Autodesk Inventor part; units mm, degrees
(part 2 of 3)
sketch "Sketch4" plane through (0, 0, -2.75) normal (0, 0, -1) x (-1, 0, 0)
  arc A0 (0.3991, 3.7387) -> (0.581, 3.8546) centre (0.3991, 3.9394) ccw
  line L0 (0.581, 3.8546) -> (0.7391, 4.1936)
  arc A1 (1.0847, 4.3585) -> (0.7391, 4.1936) centre (1.012, 4.0663) ccw
  arc A2 (1.2398, 4.317) -> (1.0847, 4.3585) centre (0, 0) ccw
  arc A3 (1.4567, 4.0013) -> (1.2398, 4.317) centre (1.1567, 4.0275) ccw
  line L1 (1.4567, 4.0013) -> (1.4241, 3.6287)
  arc A4 (1.4241, 3.6287) -> (1.5237, 3.4373) centre (1.6241, 3.6112) ccw
  line L2 (1.5237, 3.4373) -> (2.2149, 3.0382)
  arc A5 (2.2149, 3.0382) -> (2.4305, 3.0476) centre (2.3153, 3.2121) ccw
  line L3 (2.4305, 3.0476) -> (2.7369, 3.2622)
  arc A6 (3.1187, 3.2322) -> (2.7369, 3.2622) centre (2.9096, 3.0155) ccw
  arc A7 (3.2322, 3.1187) -> (3.1187, 3.2322) centre (0, 0) ccw
  arc A8 (3.2622, 2.7369) -> (3.2322, 3.1187) centre (3.0155, 2.9096) ccw
  line L4 (3.2622, 2.7369) -> (3.0476, 2.4305)
  arc A9 (3.0476, 2.4305) -> (3.0382, 2.2149) centre (3.2121, 2.3153) ccw
  line L5 (3.0382, 2.2149) -> (3.4373, 1.5237)
  arc A10 (3.4373, 1.5237) -> (3.6287, 1.4241) centre (3.6112, 1.6241) ccw
  line L6 (3.6287, 1.4241) -> (4.0013, 1.4567)
  arc A11 (4.317, 1.2398) -> (4.0013, 1.4567) centre (4.0275, 1.1567) ccw
  arc A12 (4.3585, 1.0847) -> (4.317, 1.2398) centre (0, 0) ccw
  arc A13 (4.1936, 0.7391) -> (4.3585, 1.0847) centre (4.0663, 1.012) ccw
  line L7 (4.1936, 0.7391) -> (3.8546, 0.581)
  arc A14 (3.8546, 0.581) -> (3.7387, 0.3991) centre (3.9394, 0.3991) ccw
  line L8 (3.7387, 0.3991) -> (3.7387, -0.3991)
  arc A15 (3.7387, -0.3991) -> (3.8546, -0.581) centre (3.9394, -0.3991) ccw
  line L9 (3.8546, -0.581) -> (4.1936, -0.7391)
  arc A16 (4.3585, -1.0847) -> (4.1936, -0.7391) centre (4.0663, -1.012) ccw
  arc A17 (4.317, -1.2398) -> (4.3585, -1.0847) centre (0, 0) ccw
  arc A18 (4.0013, -1.4567) -> (4.317, -1.2398) centre (4.0275, -1.1567) ccw
  line L10 (4.0013, -1.4567) -> (3.6287, -1.4241)
  arc A19 (3.6287, -1.4241) -> (3.4373, -1.5237) centre (3.6112, -1.6241) ccw
  line L11 (3.4373, -1.5237) -> (3.0382, -2.2149)
  arc A20 (3.0382, -2.2149) -> (3.0476, -2.4305) centre (3.2121, -2.3153) ccw
  line L12 (3.0476, -2.4305) -> (3.2622, -2.7369)
  arc A21 (3.2322, -3.1187) -> (3.2622, -2.7369) centre (3.0155, -2.9096) ccw
  arc A22 (3.1187, -3.2322) -> (3.2322, -3.1187) centre (0, 0) ccw
  arc A23 (2.7369, -3.2622) -> (3.1187, -3.2322) centre (2.9096, -3.0155) ccw
  line L13 (2.7369, -3.2622) -> (2.4305, -3.0476)
  arc A24 (2.4305, -3.0476) -> (2.2149, -3.0382) centre (2.3153, -3.2121) ccw
  line L14 (2.2149, -3.0382) -> (1.5237, -3.4373)
  arc A25 (1.5237, -3.4373) -> (1.4241, -3.6287) centre (1.6241, -3.6112) ccw
  line L15 (1.4241, -3.6287) -> (1.4567, -4.0013)
  arc A26 (1.2398, -4.317) -> (1.4567, -4.0013) centre (1.1567, -4.0275) ccw
  arc A27 (1.0847, -4.3585) -> (1.2398, -4.317) centre (0, 0) ccw
  arc A28 (0.7391, -4.1936) -> (1.0847, -4.3585) centre (1.012, -4.0663) ccw
  line L16 (0.7391, -4.1936) -> (0.581, -3.8546)
  arc A29 (0.581, -3.8546) -> (0.3991, -3.7387) centre (0.3991, -3.9394) ccw
  line L17 (0.3991, -3.7387) -> (-0.3991, -3.7387)
  arc A30 (-0.3991, -3.7387) -> (-0.581, -3.8546) centre (-0.3991, -3.9394) ccw
  line L18 (-0.581, -3.8546) -> (-0.7391, -4.1936)
  arc A31 (-1.0847, -4.3585) -> (-0.7391, -4.1936) centre (-1.012, -4.0663) ccw
  arc A32 (-1.2398, -4.317) -> (-1.0847, -4.3585) centre (0, 0) ccw
  arc A33 (-1.4567, -4.0013) -> (-1.2398, -4.317) centre (-1.1567, -4.0275) ccw
  line L19 (-1.4567, -4.0013) -> (-1.4241, -3.6287)
  arc A34 (-1.4241, -3.6287) -> (-1.5237, -3.4373) centre (-1.6241, -3.6112) ccw
  line L20 (-1.5237, -3.4373) -> (-2.2149, -3.0382)
  arc A35 (-2.2149, -3.0382) -> (-2.4305, -3.0476) centre (-2.3153, -3.2121) ccw
  line L21 (-2.4305, -3.0476) -> (-2.7369, -3.2622)
  arc A36 (-3.1187, -3.2322) -> (-2.7369, -3.2622) centre (-2.9096, -3.0155) ccw
  arc A37 (-3.2322, -3.1187) -> (-3.1187, -3.2322) centre (0, 0) ccw
  arc A38 (-3.2622, -2.7369) -> (-3.2322, -3.1187) centre (-3.0155, -2.9096) ccw
  line L22 (-3.2622, -2.7369) -> (-3.0476, -2.4305)
  arc A39 (-3.0476, -2.4305) -> (-3.0382, -2.2149) centre (-3.2121, -2.3153) ccw
  line L23 (-3.0382, -2.2149) -> (-3.4373, -1.5237)
  arc A40 (-3.4373, -1.5237) -> (-3.6287, -1.4241) centre (-3.6112, -1.6241) ccw
  line L24 (-3.6287, -1.4241) -> (-4.0013, -1.4567)
  arc A41 (-4.317, -1.2398) -> (-4.0013, -1.4567) centre (-4.0275, -1.1567) ccw
  arc A42 (-4.3585, -1.0847) -> (-4.317, -1.2398) centre (0, 0) ccw
  arc A43 (-4.1936, -0.7391) -> (-4.3585, -1.0847) centre (-4.0663, -1.012) ccw
  line L25 (-4.1936, -0.7391) -> (-3.8546, -0.581)
  arc A44 (-3.8546, -0.581) -> (-3.7387, -0.3991) centre (-3.9394, -0.3991) ccw
  line L26 (-3.7387, -0.3991) -> (-3.7387, 0.3991)
  arc A45 (-3.7387, 0.3991) -> (-3.8546, 0.581) centre (-3.9394, 0.3991) ccw
  line L27 (-3.8546, 0.581) -> (-4.1936, 0.7391)
  arc A46 (-4.3585, 1.0847) -> (-4.1936, 0.7391) centre (-4.0663, 1.012) ccw
  arc A47 (-4.317, 1.2398) -> (-4.3585, 1.0847) centre (0, 0) ccw
  arc A48 (-4.0013, 1.4567) -> (-4.317, 1.2398) centre (-4.0275, 1.1567) ccw
  line L28 (-4.0013, 1.4567) -> (-3.6287, 1.4241)
  arc A49 (-3.6287, 1.4241) -> (-3.4373, 1.5237) centre (-3.6112, 1.6241) ccw
  line L29 (-3.4373, 1.5237) -> (-3.0382, 2.2149)
  arc A50 (-3.0382, 2.2149) -> (-3.0476, 2.4305) centre (-3.2121, 2.3153) ccw
  line L30 (-3.0476, 2.4305) -> (-3.2622, 2.7369)
  arc A51 (-3.2322, 3.1187) -> (-3.2622, 2.7369) centre (-3.0155, 2.9096) ccw
  arc A52 (-3.1187, 3.2322) -> (-3.2322, 3.1187) centre (0, 0) ccw
  arc A53 (-2.7369, 3.2622) -> (-3.1187, 3.2322) centre (-2.9096, 3.0155) ccw
  line L31 (-2.7369, 3.2622) -> (-2.4305, 3.0476)
  arc A54 (-2.4305, 3.0476) -> (-2.2149, 3.0382) centre (-2.3153, 3.2121) ccw
  line L32 (-2.2149, 3.0382) -> (-1.5237, 3.4373)
  arc A55 (-1.5237, 3.4373) -> (-1.4241, 3.6287) centre (-1.6241, 3.6112) ccw
  line L33 (-1.4241, 3.6287) -> (-1.4567, 4.0013)
  arc A56 (-1.2398, 4.317) -> (-1.4567, 4.0013) centre (-1.1567, 4.0275) ccw
  arc A57 (-1.0847, 4.3585) -> (-1.2398, 4.317) centre (0, 0) ccw
  arc A58 (-0.7391, 4.1936) -> (-1.0847, 4.3585) centre (-1.012, 4.0663) ccw
  line L34 (-0.7391, 4.1936) -> (-0.581, 3.8546)
  arc A59 (-0.581, 3.8546) -> (-0.3991, 3.7387) centre (-0.3991, 3.9394) ccw
  line L35 (-0.3991, 3.7387) -> (0.3991, 3.7387)
  circle A60 centre (0, 0) radius 6.84
  arc A61 (3.6199, -1.5237) -> (3.5239, -1.5737) centre (3.6112, -1.6241) ccw
  circle A62 centre (0, 0) radius 4.4915 construction
  line L36 (-2.3024, -3.1898) -> (-1.6112, -3.5889)
  arc A63 (-1.5984, -3.6134) -> (-1.6112, -3.5889) centre (-1.6241, -3.6112) ccw
  line L37 (-1.5984, -3.6134) -> (-1.631, -3.986)
  arc A64 (-1.631, -3.986) -> (-1.2882, -4.4852) centre (-1.1567, -4.0275) ccw
  arc A65 (-1.2882, -4.4852) -> (-1.127, -4.5283) centre (0, 0) ccw
  arc A66 (-1.127, -4.5283) -> (-0.5805, -4.2675) centre (-1.012, -4.0663) ccw
  line L38 (-0.5805, -4.2675) -> (-0.4224, -3.9285)
  arc A67 (-0.3991, -3.9137) -> (-0.4224, -3.9285) centre (-0.3991, -3.9394) ccw
  line L39 (-0.3991, -3.9137) -> (0.3991, -3.9137)
  arc A68 (0.4224, -3.9285) -> (0.3991, -3.9137) centre (0.3991, -3.9394) ccw
  line L40 (0.4224, -3.9285) -> (0.5805, -4.2675)
  arc A69 (0.5805, -4.2675) -> (1.127, -4.5283) centre (1.012, -4.0663) ccw
  arc A70 (1.127, -4.5283) -> (1.2882, -4.4852) centre (0, 0) ccw
  arc A71 (1.2882, -4.4852) -> (1.631, -3.986) centre (1.1567, -4.0275) ccw
  line L41 (1.631, -3.986) -> (1.5984, -3.6134)
  arc A72 (1.6112, -3.5889) -> (1.5984, -3.6134) centre (1.6241, -3.6112) ccw
  line L42 (1.6112, -3.5889) -> (2.3024, -3.1898)
  arc A73 (2.3301, -3.191) -> (2.3024, -3.1898) centre (2.3153, -3.2121) ccw
  line L43 (2.3301, -3.191) -> (2.6365, -3.4055)
  arc A74 (2.6365, -3.4055) -> (3.2402, -3.3582) centre (2.9096, -3.0155) ccw
  arc A75 (3.2402, -3.3582) -> (3.3582, -3.2402) centre (0, 0) ccw
  arc A76 (3.3582, -3.2402) -> (3.4055, -2.6365) centre (3.0155, -2.9096) ccw
  line L44 (3.4055, -2.6365) -> (3.191, -2.3301)
  arc A77 (3.1898, -2.3024) -> (3.191, -2.3301) centre (3.2121, -2.3153) ccw
  line L45 (3.1898, -2.3024) -> (3.5889, -1.6112)
  arc A78 (3.6134, -1.5984) -> (3.5889, -1.6112) centre (3.6112, -1.6241) ccw
  line L46 (3.6134, -1.5984) -> (3.986, -1.631)
  arc A79 (3.986, -1.631) -> (4.4852, -1.2882) centre (4.0275, -1.1567) ccw
  arc A80 (4.4852, -1.2882) -> (4.5283, -1.127) centre (0, 0) ccw
  arc A81 (4.5283, -1.127) -> (4.2675, -0.5805) centre (4.0663, -1.012) ccw
  line L47 (4.2675, -0.5805) -> (3.9285, -0.4224)
  arc A82 (3.9137, -0.3991) -> (3.9285, -0.4224) centre (3.9394, -0.3991) ccw
  line L48 (3.9137, -0.3991) -> (3.9137, 0.3991)
  arc A83 (3.9285, 0.4224) -> (3.9137, 0.3991) centre (3.9394, 0.3991) ccw
  line L49 (3.9285, 0.4224) -> (4.2675, 0.5805)
  arc A84 (4.2675, 0.5805) -> (4.5283, 1.127) centre (4.0663, 1.012) ccw
  arc A85 (4.5283, 1.127) -> (4.4852, 1.2882) centre (0, 0) ccw
  arc A86 (4.4852, 1.2882) -> (3.986, 1.631) centre (4.0275, 1.1567) ccw
  line L50 (3.986, 1.631) -> (3.6134, 1.5984)
  arc A87 (3.5889, 1.6112) -> (3.6134, 1.5984) centre (3.6112, 1.6241) ccw
  line L51 (3.5889, 1.6112) -> (3.1898, 2.3024)
  arc A88 (3.191, 2.3301) -> (3.1898, 2.3024) centre (3.2121, 2.3153) ccw
  line L52 (3.191, 2.3301) -> (3.4055, 2.6365)
  arc A89 (3.4055, 2.6365) -> (3.3582, 3.2402) centre (3.0155, 2.9096) ccw
  arc A90 (3.3582, 3.2402) -> (3.2402, 3.3582) centre (0, 0) ccw
  arc A91 (3.2402, 3.3582) -> (2.6365, 3.4055) centre (2.9096, 3.0155) ccw
  line L53 (2.6365, 3.4055) -> (2.3301, 3.191)
  arc A92 (2.3024, 3.1898) -> (2.3301, 3.191) centre (2.3153, 3.2121) ccw
  line L54 (2.3024, 3.1898) -> (1.6112, 3.5889)
  arc A93 (1.5984, 3.6134) -> (1.6112, 3.5889) centre (1.6241, 3.6112) ccw
  line L55 (1.5984, 3.6134) -> (1.631, 3.986)
  arc A94 (1.631, 3.986) -> (1.2882, 4.4852) centre (1.1567, 4.0275) ccw
  arc A95 (1.2882, 4.4852) -> (1.127, 4.5283) centre (0, 0) ccw
  arc A96 (1.127, 4.5283) -> (0.5805, 4.2675) centre (1.012, 4.0663) ccw
  line L56 (0.5805, 4.2675) -> (0.4224, 3.9285)
  arc A97 (0.3991, 3.9137) -> (0.4224, 3.9285) centre (0.3991, 3.9394) ccw
  line L57 (0.3991, 3.9137) -> (-0.3991, 3.9137)
  arc A98 (-0.4224, 3.9285) -> (-0.3991, 3.9137) centre (-0.3991, 3.9394) ccw
  line L58 (-0.4224, 3.9285) -> (-0.5805, 4.2675)
  arc A99 (-0.5805, 4.2675) -> (-1.127, 4.5283) centre (-1.012, 4.0663) ccw
  arc A100 (-1.127, 4.5283) -> (-1.2882, 4.4852) centre (0, 0) ccw
  arc A101 (-1.2882, 4.4852) -> (-1.631, 3.986) centre (-1.1567, 4.0275) ccw
  line L59 (-1.631, 3.986) -> (-1.5984, 3.6134)
  arc A102 (-1.6112, 3.5889) -> (-1.5984, 3.6134) centre (-1.6241, 3.6112) ccw
  line L60 (-1.6112, 3.5889) -> (-2.3024, 3.1898)
  arc A103 (-2.3301, 3.191) -> (-2.3024, 3.1898) centre (-2.3153, 3.2121) ccw
  line L61 (-2.3301, 3.191) -> (-2.6365, 3.4055)
  arc A104 (-2.6365, 3.4055) -> (-3.2402, 3.3582) centre (-2.9096, 3.0155) ccw
  arc A105 (-3.2402, 3.3582) -> (-3.3582, 3.2402) centre (0, 0) ccw
  arc A106 (-3.3582, 3.2402) -> (-3.4055, 2.6365) centre (-3.0155, 2.9096) ccw
  line L62 (-3.4055, 2.6365) -> (-3.191, 2.3301)
  arc A107 (-3.1898, 2.3024) -> (-3.191, 2.3301) centre (-3.2121, 2.3153) ccw
  line L63 (-3.1898, 2.3024) -> (-3.5889, 1.6112)
  arc A108 (-3.6134, 1.5984) -> (-3.5889, 1.6112) centre (-3.6112, 1.6241) ccw
  line L64 (-3.6134, 1.5984) -> (-3.986, 1.631)
  arc A109 (-3.986, 1.631) -> (-4.4852, 1.2882) centre (-4.0275, 1.1567) ccw
  arc A110 (-4.4852, 1.2882) -> (-4.5283, 1.127) centre (0, 0) ccw
  arc A111 (-4.5283, 1.127) -> (-4.2675, 0.5805) centre (-4.0663, 1.012) ccw
  line L65 (-4.2675, 0.5805) -> (-3.9285, 0.4224)
  arc A112 (-3.9137, 0.3991) -> (-3.9285, 0.4224) centre (-3.9394, 0.3991) ccw
  line L66 (-3.9137, 0.3991) -> (-3.9137, -0.3991)
  arc A113 (-3.9285, -0.4224) -> (-3.9137, -0.3991) centre (-3.9394, -0.3991) ccw
  line L67 (-3.9285, -0.4224) -> (-4.2675, -0.5805)
  arc A114 (-4.2675, -0.5805) -> (-4.5283, -1.127) centre (-4.0663, -1.012) ccw
  arc A115 (-4.5283, -1.127) -> (-4.4852, -1.2882) centre (0, 0) ccw
  arc A116 (-4.4852, -1.2882) -> (-3.986, -1.631) centre (-4.0275, -1.1567) ccw
  line L68 (-3.986, -1.631) -> (-3.6134, -1.5984)
  arc A117 (-3.5889, -1.6112) -> (-3.6134, -1.5984) centre (-3.6112, -1.6241) ccw
  line L69 (-3.5889, -1.6112) -> (-3.1898, -2.3024)
  arc A118 (-3.191, -2.3301) -> (-3.1898, -2.3024) centre (-3.2121, -2.3153) ccw
  line L70 (-3.191, -2.3301) -> (-3.4055, -2.6365)
  arc A119 (-3.4055, -2.6365) -> (-3.3582, -3.2402) centre (-3.0155, -2.9096) ccw
  arc A120 (-3.3582, -3.2402) -> (-3.2402, -3.3582) centre (0, 0) ccw
  arc A121 (-3.2402, -3.3582) -> (-2.6365, -3.4055) centre (-2.9096, -3.0155) ccw
  line L71 (-2.6365, -3.4055) -> (-2.3301, -3.191)
  arc A122 (-2.3024, -3.1898) -> (-2.3301, -3.191) centre (-2.3153, -3.2121) ccw
  dimension "d0" = 28.6479
  dimension "d1" = 0.3
  dimension "d2" = 0.75
  dimension "d3" = 50
  dimension "d4" = 1.05
  dimension "d74" = 8.983
  dimension "d34" = 13.68
  dimension "d75" = 0.175
  constraints: 242 point on circle, 144 end point, 122 centre point, 3 coincident, 98 other
  measures "d34" diameter of A60
  measures "d75" distance between parallel lines of L20 L36
sketch "HTD3M 33Teeth" plane through (0, 0, 0) normal (0, 0, 1) x (1, 0, 0)
  arc A0 (15.2288, 2.1154) -> (15.2079, 2.2607) centre (0, 0) ccw
  arc A1 (15.1485, 1.9322) -> (15.2288, 2.1154) centre (15.0396, 2.0891) ccw
  line L0 (15.1485, 1.9322) -> (14.5361, 1.5072)
  arc A2 (14.5361, 1.5072) -> (14.1386, 0.7015) centre (15.0646, 0.7456) ccw
  line L1 (14.1386, 0.7015) -> (14.1413, 0.6456)
  arc A3 (14.1413, 0.6456) -> (14.6135, -0.1187) centre (15.0672, 0.6897) ccw
  line L2 (14.6135, -0.1187) -> (15.2636, -0.4835)
  arc A4 (15.3609, -0.6583) -> (15.2636, -0.4835) centre (15.1701, -0.6501) ccw
  arc A5 (15.3539, -0.8049) -> (15.3609, -0.6583) centre (0, 0) ccw
  arc A6 (15.2404, -0.9696) -> (15.3539, -0.8049) centre (15.1632, -0.7949) ccw
  line L3 (15.2404, -0.9696) -> (14.5586, -1.271)
  arc A7 (14.5586, -1.271) -> (14.0159, -1.9869) centre (14.9335, -2.1188) ccw
  line L4 (14.0159, -1.9869) -> (14.0079, -2.0423)
  arc A8 (14.0079, -2.0423) -> (14.327, -2.8821) centre (14.9255, -2.1742) ccw
  line L5 (14.327, -2.8821) -> (14.8962, -3.3634)
  arc A9 (14.9587, -3.5534) -> (14.8962, -3.3634) centre (14.7729, -3.5093) ccw
  arc A10 (14.9241, -3.6961) -> (14.9587, -3.5534) centre (0, 0) ccw
  arc A11 (14.7815, -3.8363) -> (14.9241, -3.6961) centre (14.7387, -3.6502) ccw
  line L6 (14.7815, -3.8363) -> (14.055, -4.0033)
  arc A12 (14.055, -4.0033) -> (13.3866, -4.6035) centre (14.2626, -4.9067) ccw
  line L7 (13.3866, -4.6035) -> (13.3683, -4.6564)
  arc A13 (13.3683, -4.6564) -> (13.5226, -5.5415) centre (14.2443, -4.9596) ccw
  line L8 (13.5226, -5.5415) -> (13.9905, -6.1218)
  arc A14 (14.0159, -6.3202) -> (13.9905, -6.1218) centre (13.8418, -6.2417) ccw
  arc A15 (13.9549, -6.4537) -> (14.0159, -6.3202) centre (0, 0) ccw
  arc A16 (13.7884, -6.5644) -> (13.9549, -6.4537) centre (13.7816, -6.3735) ccw
  line L9 (13.7884, -6.5644) -> (13.0434, -6.5908)
  arc A17 (13.0434, -6.5908) -> (12.2735, -7.0538) centre (13.0763, -7.5173) ccw
  line L10 (12.2735, -7.0538) -> (12.2455, -7.1022)
  arc A18 (12.2455, -7.1022) -> (12.2295, -8.0005) centre (13.0483, -7.5657) ccw
  line L11 (12.2295, -8.0005) -> (12.5791, -8.6589)
  arc A19 (12.5665, -8.8585) -> (12.5791, -8.6589) centre (12.4104, -8.7484) ccw
  arc A20 (12.4814, -8.9781) -> (12.5665, -8.8585) centre (0, 0) ccw
  arc A21 (12.2969, -9.0552) -> (12.4814, -8.9781) centre (12.3263, -8.8665) ccw
  line L12 (12.2969, -9.0552) -> (11.5604, -8.9402)
  arc A22 (11.5604, -8.9402) -> (10.7167, -9.249) centre (11.4173, -9.8561) ccw
  line L13 (10.7167, -9.249) -> (10.6801, -9.2914)
  arc A23 (10.6801, -9.2914) -> (10.4944, -10.1704) centre (11.3806, -9.8984) ccw
  line L14 (10.4944, -10.1704) -> (10.7131, -10.883)
  arc A24 (10.663, -11.0766) -> (10.7131, -10.883) centre (10.5305, -10.939) ccw
  arc A25 (10.5567, -11.1779) -> (10.663, -11.0766) centre (0, 0) ccw
  arc A26 (10.3609, -11.2188) -> (10.5567, -11.1779) centre (10.4256, -11.0391) ccw
  line L15 (10.3609, -11.2188) -> (9.6595, -10.9665)
  arc A27 (9.6595, -10.9665) -> (8.7727, -11.1101) centre (9.3457, -11.8387) ccw
  line L16 (8.7727, -11.1101) -> (8.7286, -11.1447)
  arc A28 (8.7286, -11.1447) -> (8.38, -11.9726) centre (9.3017, -11.8733) ccw
  line L17 (8.38, -11.9726) -> (8.4599, -12.7138)
  arc A29 (8.374, -12.8944) -> (8.4599, -12.7138) centre (8.27, -12.7343) ccw
  arc A30 (8.2505, -12.9738) -> (8.374, -12.8944) centre (0, 0) ccw
  arc A31 (8.0505, -12.9769) -> (8.2505, -12.9738) centre (8.148, -12.8126) ccw
  line L18 (8.0505, -12.9769) -> (7.4095, -12.5963)
  arc A32 (7.4095, -12.5963) -> (6.5115, -12.5695) centre (6.9363, -13.3935) ccw
  line L19 (6.5115, -12.5695) -> (6.4618, -12.5952)
  arc A33 (6.4618, -12.5952) -> (5.9627, -13.3422) centre (6.8865, -13.4191) ccw
  line L20 (5.9627, -13.3422) -> (5.9009, -14.0851)
  arc A34 (5.7824, -14.2462) -> (5.9009, -14.0851) centre (5.7105, -14.0692) ccw
  arc A35 (5.6461, -14.3008) -> (5.7824, -14.2462) centre (0, 0) ccw
  arc A36 (5.4492, -14.2659) -> (5.6461, -14.3008) centre (5.576, -14.1231) ccw
  line L21 (5.4492, -14.2659) -> (4.8917, -13.771)
  arc A37 (4.8917, -13.771) -> (4.0151, -13.5747) centre (4.2762, -14.4641) ccw
  line L22 (4.0151, -13.5747) -> (3.9613, -13.5905)
  arc A38 (3.9613, -13.5905) -> (3.33, -14.2296) centre (4.2225, -14.4799) ccw
  line L23 (3.33, -14.2296) -> (3.1286, -14.9473)
  arc A39 (2.9818, -15.0831) -> (3.1286, -14.9473) centre (2.9447, -14.8957) ccw
  arc A40 (2.8376, -15.1109) -> (2.9818, -15.0831) centre (0, 0) ccw
  arc A41 (2.6508, -15.0394) -> (2.8376, -15.1109) centre (2.8024, -14.9232) ccw
  line L24 (2.6508, -15.0394) -> (2.1972, -14.4479)
  arc A42 (2.1972, -14.4479) -> (1.3735, -14.0892) centre (1.4616, -15.012) ccw
  line L25 (1.3735, -14.0892) -> (1.3177, -14.0946)
  arc A43 (1.3177, -14.0946) -> (0.5768, -14.6026) centre (1.4059, -15.0174) ccw
  line L26 (0.5768, -14.6026) -> (0.2433, -15.2693)
  arc A44 (0.0734, -15.3748) -> (0.2433, -15.2693) centre (0.0725, -15.1838) ccw
  arc A45 (-0.0734, -15.3748) -> (0.0734, -15.3748) centre (0, 0) ccw
  arc A46 (-0.2433, -15.2693) -> (-0.0734, -15.3748) centre (-0.0725, -15.1838) ccw
  line L27 (-0.2433, -15.2693) -> (-0.5768, -14.6026)
  arc A47 (-0.5768, -14.6026) -> (-1.3177, -14.0946) centre (-1.4059, -15.0174) ccw
  line L28 (-1.3177, -14.0946) -> (-1.3735, -14.0892)
  arc A48 (-1.3735, -14.0892) -> (-2.1972, -14.4479) centre (-1.4616, -15.012) ccw
  line L29 (-2.1972, -14.4479) -> (-2.6508, -15.0394)
  arc A49 (-2.8376, -15.1109) -> (-2.6508, -15.0394) centre (-2.8024, -14.9232) ccw
  arc A50 (-2.9818, -15.0831) -> (-2.8376, -15.1109) centre (0, 0) ccw
  arc A51 (-3.1286, -14.9473) -> (-2.9818, -15.0831) centre (-2.9447, -14.8957) ccw
  line L30 (-3.1286, -14.9473) -> (-3.33, -14.2296)
  arc A52 (-3.33, -14.2296) -> (-3.9613, -13.5905) centre (-4.2225, -14.4799) ccw
  line L31 (-3.9613, -13.5905) -> (-4.0151, -13.5747)
  arc A53 (-4.0151, -13.5747) -> (-4.8917, -13.771) centre (-4.2762, -14.4641) ccw
  line L32 (-4.8917, -13.771) -> (-5.4492, -14.2659)
  arc A54 (-5.6461, -14.3008) -> (-5.4492, -14.2659) centre (-5.576, -14.1231) ccw
  arc A55 (-5.7824, -14.2462) -> (-5.6461, -14.3008) centre (0, 0) ccw
  arc A56 (-5.9009, -14.0851) -> (-5.7824, -14.2462) centre (-5.7105, -14.0692) ccw
  line L33 (-5.9009, -14.0851) -> (-5.9627, -13.3422)
  arc A57 (-5.9627, -13.3422) -> (-6.4618, -12.5952) centre (-6.8865, -13.4191) ccw
  line L34 (-6.4618, -12.5952) -> (-6.5115, -12.5695)
  arc A58 (-6.5115, -12.5695) -> (-7.4095, -12.5963) centre (-6.9363, -13.3935) ccw
  line L35 (-7.4095, -12.5963) -> (-8.0505, -12.9769)
  arc A59 (-8.2505, -12.9738) -> (-8.0505, -12.9769) centre (-8.148, -12.8126) ccw
  arc A60 (-8.374, -12.8944) -> (-8.2505, -12.9738) centre (0, 0) ccw
  arc A61 (-8.4599, -12.7138) -> (-8.374, -12.8944) centre (-8.27, -12.7343) ccw
  line L36 (-8.4599, -12.7138) -> (-8.38, -11.9726)
  arc A62 (-8.38, -11.9726) -> (-8.7286, -11.1447) centre (-9.3017, -11.8733) ccw
  line L37 (-8.7286, -11.1447) -> (-8.7727, -11.1101)
  arc A63 (-8.7727, -11.1101) -> (-9.6595, -10.9665) centre (-9.3457, -11.8387) ccw
  line L38 (-9.6595, -10.9665) -> (-10.3609, -11.2188)
  arc A64 (-10.5567, -11.1779) -> (-10.3609, -11.2188) centre (-10.4256, -11.0391) ccw
  arc A65 (-10.663, -11.0766) -> (-10.5567, -11.1779) centre (0, 0) ccw
  arc A66 (-10.7131, -10.883) -> (-10.663, -11.0766) centre (-10.5305, -10.939) ccw
  line L39 (-10.7131, -10.883) -> (-10.4944, -10.1704)
  arc A67 (-10.4944, -10.1704) -> (-10.6801, -9.2914) centre (-11.3806, -9.8984) ccw
  line L40 (-10.6801, -9.2914) -> (-10.7167, -9.249)
  arc A68 (-10.7167, -9.249) -> (-11.5604, -8.9402) centre (-11.4173, -9.8561) ccw
  line L41 (-11.5604, -8.9402) -> (-12.2969, -9.0552)
  arc A69 (-12.4814, -8.9781) -> (-12.2969, -9.0552) centre (-12.3263, -8.8665) ccw
  arc A70 (-12.5665, -8.8585) -> (-12.4814, -8.9781) centre (0, 0) ccw
  arc A71 (-12.5791, -8.6589) -> (-12.5665, -8.8585) centre (-12.4104, -8.7484) ccw
  line L42 (-12.5791, -8.6589) -> (-12.2295, -8.0005)
  arc A72 (-12.2295, -8.0005) -> (-12.2455, -7.1022) centre (-13.0483, -7.5657) ccw
  line L43 (-12.2455, -7.1022) -> (-12.2735, -7.0538)
  arc A73 (-12.2735, -7.0538) -> (-13.0434, -6.5908) centre (-13.0763, -7.5173) ccw
  line L44 (-13.0434, -6.5908) -> (-13.7884, -6.5644)
  arc A74 (-13.9549, -6.4537) -> (-13.7884, -6.5644) centre (-13.7816, -6.3735) ccw
  arc A75 (-14.0159, -6.3202) -> (-13.9549, -6.4537) centre (0, 0) ccw
  arc A76 (-13.9905, -6.1218) -> (-14.0159, -6.3202) centre (-13.8418, -6.2417) ccw
  line L45 (-13.9905, -6.1218) -> (-13.5226, -5.5415)
  arc A77 (-13.5226, -5.5415) -> (-13.3683, -4.6564) centre (-14.2443, -4.9596) ccw
  line L46 (-13.3683, -4.6564) -> (-13.3866, -4.6035)
  arc A78 (-13.3866, -4.6035) -> (-14.055, -4.0033) centre (-14.2626, -4.9067) ccw
  line L47 (-14.055, -4.0033) -> (-14.7815, -3.8363)
  arc A79 (-14.9241, -3.6961) -> (-14.7815, -3.8363) centre (-14.7387, -3.6502) ccw
  arc A80 (-14.9587, -3.5534) -> (-14.9241, -3.6961) centre (0, 0) ccw
  arc A81 (-14.8962, -3.3634) -> (-14.9587, -3.5534) centre (-14.7729, -3.5093) ccw
  line L48 (-14.8962, -3.3634) -> (-14.327, -2.8821)
  arc A82 (-14.327, -2.8821) -> (-14.0079, -2.0423) centre (-14.9255, -2.1742) ccw
  line L49 (-14.0079, -2.0423) -> (-14.0159, -1.9869)
  arc A83 (-14.0159, -1.9869) -> (-14.5586, -1.271) centre (-14.9335, -2.1188) ccw
  line L50 (-14.5586, -1.271) -> (-15.2404, -0.9696)
  arc A84 (-15.3539, -0.8049) -> (-15.2404, -0.9696) centre (-15.1632, -0.7949) ccw
  arc A85 (-15.3609, -0.6583) -> (-15.3539, -0.8049) centre (0, 0) ccw
  arc A86 (-15.2636, -0.4835) -> (-15.3609, -0.6583) centre (-15.1701, -0.6501) ccw
  line L51 (-15.2636, -0.4835) -> (-14.6135, -0.1187)
  arc A87 (-14.6135, -0.1187) -> (-14.1413, 0.6456) centre (-15.0672, 0.6897) ccw
  line L52 (-14.1413, 0.6456) -> (-14.1386, 0.7015)
  arc A88 (-14.1386, 0.7015) -> (-14.5361, 1.5072) centre (-15.0646, 0.7456) ccw
  line L53 (-14.5361, 1.5072) -> (-15.1485, 1.9322)
  arc A89 (-15.2288, 2.1154) -> (-15.1485, 1.9322) centre (-15.0396, 2.0891) ccw
  arc A90 (-15.2079, 2.2607) -> (-15.2288, 2.1154) centre (0, 0) ccw
  arc A91 (-15.0792, 2.4139) -> (-15.2079, 2.2607) centre (-15.019, 2.2326) ccw
  line L54 (-15.0792, 2.4139) -> (-14.3719, 2.6491)
  arc A92 (-14.3719, 2.6491) -> (-13.7636, 3.3102) centre (-14.6644, 3.5287) ccw
  line L55 (-13.7636, 3.3102) -> (-13.7504, 3.3646)
  arc A93 (-13.7504, 3.3646) -> (-13.9881, 4.231) centre (-14.6512, 3.5832) ccw
  line L56 (-13.9881, 4.231) -> (-14.5091, 4.7642)
  arc A94 (-14.5532, 4.9593) -> (-14.5091, 4.7642) centre (-14.3724, 4.8977) ccw
  arc A95 (-14.5052, 5.098) -> (-14.5532, 4.9593) centre (0, 0) ccw
  arc A96 (-14.3499, 5.224) -> (-14.5052, 5.098) centre (-14.325, 5.0346) ccw
  line L57 (-14.3499, 5.224) -> (-13.6108, 5.3211)
  arc A97 (-13.6108, 5.3211) -> (-12.8884, 5.8551) centre (-13.7316, 6.2402) ccw
  line L58 (-12.8884, 5.8551) -> (-12.8651, 5.9061)
  arc A98 (-12.8651, 5.9061) -> (-12.9346, 6.8018) centre (-13.7083, 6.2912) ccw
  line L59 (-12.9346, 6.8018) -> (-13.3452, 7.4239)
  arc A99 (-13.3517, 7.6239) -> (-13.3452, 7.4239) centre (-13.1858, 7.5291) ccw
  arc A100 (-13.2783, 7.751) -> (-13.3517, 7.6239) centre (0, 0) ccw
  arc A101 (-13.1019, 7.8453) -> (-13.2783, 7.751) centre (-13.1133, 7.6547) ccw
  line L60 (-13.1019, 7.8453) -> (-12.3578, 7.8008)
  arc A102 (-12.3578, 7.8008) -> (-11.5474, 8.1885) centre (-12.3025, 8.7262) ccw
  line L61 (-11.5474, 8.1885) -> (-11.5149, 8.2341)
  arc A103 (-11.5149, 8.2341) -> (-11.4137, 9.1267) centre (-12.27, 8.7718) ccw
  line L62 (-11.4137, 9.1267) -> (-11.6991, 9.8154)
  arc A104 (-11.6676, 10.0129) -> (-11.6991, 9.8154) centre (-11.5226, 9.8885) ccw
  arc A105 (-11.5715, 10.1238) -> (-11.6676, 10.0129) centre (0, 0) ccw
  arc A106 (-11.3804, 10.1831) -> (-11.5715, 10.1238) centre (-11.4277, 9.9981) ccw
  line L63 (-11.3804, 10.1831) -> (-10.6582, 9.9986)
  arc A107 (-10.6582, 9.9986) -> (-9.789, 10.2259) centre (-10.4287, 10.8968) ccw
  line L64 (-9.789, 10.2259) -> (-9.7485, 10.2645)
  arc A108 (-9.7485, 10.2645) -> (-9.4801, 11.1219) centre (-10.3882, 10.9354) ccw
  line L65 (-9.4801, 11.1219) -> (-9.6301, 11.8521)
  arc A109 (-9.5618, 12.0401) -> (-9.6301, 11.8521) centre (-9.443, 11.8905) ccw
  arc A110 (-9.4464, 12.1308) -> (-9.5618, 12.0401) centre (0, 0) ccw
  arc A111 (-9.2476, 12.1529) -> (-9.4464, 12.1308) centre (-9.329, 11.9801) ccw
  line L66 (-9.2476, 12.1529) -> (-8.5733, 11.835)
  arc A112 (-8.5733, 11.835) -> (-7.6769, 11.8936) centre (-8.178, 12.6735) ccw
  line L67 (-7.6769, 11.8936) -> (-7.6298, 11.9239)
  arc A113 (-7.6298, 11.9239) -> (-7.204, 12.715) centre (-8.1309, 12.7038) ccw
  line L68 (-7.204, 12.715) -> (-7.213, 13.4604)
  arc A114 (-7.1104, 13.6321) -> (-7.213, 13.4604) centre (-7.0221, 13.4627) ccw
  arc A115 (-6.9799, 13.6993) -> (-7.1104, 13.6321) centre (0, 0) ccw
  arc A116 (-6.7805, 13.6834) -> (-6.9799, 13.6993) centre (-6.8932, 13.5291) ccw
  line L69 (-6.7805, 13.6834) -> (-6.1786, 13.2436)
  arc A117 (-6.1786, 13.2436) -> (-5.2872, 13.1316) centre (-5.6318, 13.9922) ccw
  line L70 (-5.2872, 13.1316) -> (-5.2353, 13.1524)
  arc A118 (-5.2353, 13.1524) -> (-4.6675, 13.8486) centre (-5.5798, 14.013) ccw
  line L71 (-4.6675, 13.8486) -> (-4.5353, 14.5822)
  arc A119 (-4.402, 14.7314) -> (-4.5353, 14.5822) centre (-4.3473, 14.5484) ccw
  arc A120 (-4.2612, 14.7727) -> (-4.402, 14.7314) centre (0, 0) ccw
  arc A121 (-4.0684, 14.7193) -> (-4.2612, 14.7727) centre (-4.2082, 14.5892) ccw
  line L72 (-4.0684, 14.7193) -> (-3.5606, 14.1736)
  arc A122 (-3.5606, 14.1736) -> (-2.7065, 13.8949) centre (-2.882, 14.8051) ccw
  line L73 (-2.7065, 13.8949) -> (-2.6515, 13.9055)
  arc A123 (-2.6515, 13.9055) -> (-1.9623, 14.4817) centre (-2.827, 14.8157) ccw
  line L74 (-1.9623, 14.4817) -> (-1.6936, 15.177)
  arc A124 (-1.5345, 15.2982) -> (-1.6936, 15.177) centre (-1.5155, 15.1082) ccw
  arc A125 (-1.3884, 15.3122) -> (-1.5345, 15.2982) centre (0, 0) ccw
  arc A126 (-1.2092, 15.2233) -> (-1.3884, 15.3122) centre (-1.3712, 15.122) ccw
  line L75 (-1.2092, 15.2233) -> (-0.8139, 14.5913)
  arc A127 (-0.8139, 14.5913) -> (-0.028, 14.156) centre (-0.028, 15.083) ccw
  line L76 (-0.028, 14.156) -> (0.028, 14.156)
  arc A128 (0.028, 14.156) -> (0.8139, 14.5913) centre (0.028, 15.083) ccw
  line L77 (0.8139, 14.5913) -> (1.2092, 15.2233)
  arc A129 (1.3884, 15.3122) -> (1.2092, 15.2233) centre (1.3712, 15.122) ccw
  arc A130 (1.5345, 15.2982) -> (1.3884, 15.3122) centre (0, 0) ccw
  arc A131 (1.6936, 15.177) -> (1.5345, 15.2982) centre (1.5155, 15.1082) ccw
  line L78 (1.6936, 15.177) -> (1.9623, 14.4817)
  arc A132 (1.9623, 14.4817) -> (2.6515, 13.9055) centre (2.827, 14.8157) ccw
  line L79 (2.6515, 13.9055) -> (2.7065, 13.8949)
  arc A133 (2.7065, 13.8949) -> (3.5606, 14.1736) centre (2.882, 14.8051) ccw
  line L80 (3.5606, 14.1736) -> (4.0684, 14.7193)
  arc A134 (4.2612, 14.7727) -> (4.0684, 14.7193) centre (4.2082, 14.5892) ccw
  arc A135 (4.402, 14.7314) -> (4.2612, 14.7727) centre (0, 0) ccw
  arc A136 (4.5353, 14.5822) -> (4.402, 14.7314) centre (4.3473, 14.5484) ccw
  line L81 (4.5353, 14.5822) -> (4.6675, 13.8486)
  arc A137 (4.6675, 13.8486) -> (5.2353, 13.1524) centre (5.5798, 14.013) ccw
  line L82 (5.2353, 13.1524) -> (5.2872, 13.1316)
  arc A138 (5.2872, 13.1316) -> (6.1786, 13.2436) centre (5.6318, 13.9922) ccw
  line L83 (6.1786, 13.2436) -> (6.7805, 13.6834)
  arc A139 (6.9799, 13.6993) -> (6.7805, 13.6834) centre (6.8932, 13.5291) ccw
  arc A140 (7.1104, 13.6321) -> (6.9799, 13.6993) centre (0, 0) ccw
  arc A141 (7.213, 13.4604) -> (7.1104, 13.6321) centre (7.0221, 13.4627) ccw
  line L84 (7.213, 13.4604) -> (7.204, 12.715)
  arc A142 (7.204, 12.715) -> (7.6298, 11.9239) centre (8.1309, 12.7038) ccw
  line L85 (7.6298, 11.9239) -> (7.6769, 11.8936)
  arc A143 (7.6769, 11.8936) -> (8.5733, 11.835) centre (8.178, 12.6735) ccw
  line L86 (8.5733, 11.835) -> (9.2476, 12.1529)
  arc A144 (9.4464, 12.1308) -> (9.2476, 12.1529) centre (9.329, 11.9801) ccw
  arc A145 (9.5618, 12.0401) -> (9.4464, 12.1308) centre (0, 0) ccw
  arc A146 (9.6301, 11.8521) -> (9.5618, 12.0401) centre (9.443, 11.8905) ccw
  line L87 (9.6301, 11.8521) -> (9.4801, 11.1219)
  arc A147 (9.4801, 11.1219) -> (9.7485, 10.2645) centre (10.3882, 10.9354) ccw
  line L88 (9.7485, 10.2645) -> (9.789, 10.2259)
  arc A148 (9.789, 10.2259) -> (10.6582, 9.9986) centre (10.4287, 10.8968) ccw
  line L89 (10.6582, 9.9986) -> (11.3804, 10.1831)
  arc A149 (11.5715, 10.1238) -> (11.3804, 10.1831) centre (11.4277, 9.9981) ccw
  arc A150 (11.6676, 10.0129) -> (11.5715, 10.1238) centre (0, 0) ccw
  arc A151 (11.6991, 9.8154) -> (11.6676, 10.0129) centre (11.5226, 9.8885) ccw
  line L90 (11.6991, 9.8154) -> (11.4137, 9.1267)
  arc A152 (11.4137, 9.1267) -> (11.5149, 8.2341) centre (12.27, 8.7718) ccw
  line L91 (11.5149, 8.2341) -> (11.5474, 8.1885)
  arc A153 (11.5474, 8.1885) -> (12.3578, 7.8008) centre (12.3025, 8.7262) ccw
  line L92 (12.3578, 7.8008) -> (13.1019, 7.8453)
  arc A154 (13.2783, 7.751) -> (13.1019, 7.8453) centre (13.1133, 7.6547) ccw
  arc A155 (13.3517, 7.6239) -> (13.2783, 7.751) centre (0, 0) ccw
  arc A156 (13.3452, 7.4239) -> (13.3517, 7.6239) centre (13.1858, 7.5291) ccw
  line L93 (13.3452, 7.4239) -> (12.9346, 6.8018)
  arc A157 (12.9346, 6.8018) -> (12.8651, 5.9061) centre (13.7083, 6.2912) ccw
  line L94 (12.8651, 5.9061) -> (12.8884, 5.8551)
  arc A158 (12.8884, 5.8551) -> (13.6108, 5.3211) centre (13.7316, 6.2402) ccw
  line L95 (13.6108, 5.3211) -> (14.3499, 5.224)
  arc A159 (14.5052, 5.098) -> (14.3499, 5.224) centre (14.325, 5.0346) ccw
  arc A160 (14.5532, 4.9593) -> (14.5052, 5.098) centre (0, 0) ccw
  arc A161 (14.5091, 4.7642) -> (14.5532, 4.9593) centre (14.3724, 4.8977) ccw
  line L96 (14.5091, 4.7642) -> (13.9881, 4.231)
  arc A162 (13.9881, 4.231) -> (13.7504, 3.3646) centre (14.6512, 3.5832) ccw
  line L97 (13.7504, 3.3646) -> (13.7636, 3.3102)
  arc A163 (13.7636, 3.3102) -> (14.3719, 2.6491) centre (14.6644, 3.5287) ccw
  line L98 (14.3719, 2.6491) -> (15.0792, 2.4139)
  arc A164 (15.2079, 2.2607) -> (15.0792, 2.4139) centre (15.019, 2.2326) ccw
  arc A165 (15.2288, 2.1154) -> (15.2079, 2.2607) centre (0, 0) ccw
  arc A166 (15.1485, 1.9322) -> (15.2288, 2.1154) centre (15.0396, 2.0891) ccw
  line L99 (15.1485, 1.9322) -> (14.5361, 1.5072)
  arc A167 (14.5361, 1.5072) -> (14.1386, 0.7015) centre (15.0646, 0.7456) ccw
  line L100 (14.1386, 0.7015) -> (14.1413, 0.6456)
  arc A168 (14.1413, 0.6456) -> (14.6135, -0.1187) centre (15.0672, 0.6897) ccw
  line L101 (14.6135, -0.1187) -> (15.2636, -0.4835)
  arc A169 (15.3609, -0.6583) -> (15.2636, -0.4835) centre (15.1701, -0.6501) ccw
  arc A170 (15.3539, -0.8049) -> (15.3609, -0.6583) centre (0, 0) ccw
  arc A171 (15.2404, -0.9696) -> (15.3539, -0.8049) centre (15.1632, -0.7949) ccw
  line L102 (15.2404, -0.9696) -> (14.5586, -1.271)
  arc A172 (14.5586, -1.271) -> (14.0159, -1.9869) centre (14.9335, -2.1188) ccw
  line L103 (14.0159, -1.9869) -> (14.0079, -2.0423)
  arc A173 (14.0079, -2.0423) -> (14.327, -2.8821) centre (14.9255, -2.1742) ccw
  line L104 (14.327, -2.8821) -> (14.8962, -3.3634)
  arc A174 (14.9587, -3.5534) -> (14.8962, -3.3634) centre (14.7729, -3.5093) ccw
  arc A175 (14.9241, -3.6961) -> (14.9587, -3.5534) centre (0, 0) ccw
  arc A176 (14.7815, -3.8363) -> (14.9241, -3.6961) centre (14.7387, -3.6502) ccw
  line L105 (14.7815, -3.8363) -> (14.055, -4.0033)
  arc A177 (14.055, -4.0033) -> (13.3866, -4.6035) centre (14.2626, -4.9067) ccw
  line L106 (13.3866, -4.6035) -> (13.3683, -4.6564)
  arc A178 (13.3683, -4.6564) -> (13.5226, -5.5415) centre (14.2443, -4.9596) ccw
  line L107 (13.5226, -5.5415) -> (13.9905, -6.1218)
  arc A179 (14.0159, -6.3202) -> (13.9905, -6.1218) centre (13.8418, -6.2417) ccw
  arc A180 (13.9549, -6.4537) -> (14.0159, -6.3202) centre (0, 0) ccw
  arc A181 (13.7884, -6.5644) -> (13.9549, -6.4537) centre (13.7816, -6.3735) ccw
  line L108 (13.7884, -6.5644) -> (13.0434, -6.5908)
  arc A182 (13.0434, -6.5908) -> (12.2735, -7.0538) centre (13.0763, -7.5173) ccw
  line L109 (12.2735, -7.0538) -> (12.2455, -7.1022)
  arc A183 (12.2455, -7.1022) -> (12.2295, -8.0005) centre (13.0483, -7.5657) ccw
  line L110 (12.2295, -8.0005) -> (12.5791, -8.6589)
  arc A184 (12.5665, -8.8585) -> (12.5791, -8.6589) centre (12.4104, -8.7484) ccw
  arc A185 (12.4814, -8.9781) -> (12.5665, -8.8585) centre (0, 0) ccw
  arc A186 (12.2969, -9.0552) -> (12.4814, -8.9781) centre (12.3263, -8.8665) ccw
  line L111 (12.2969, -9.0552) -> (11.5604, -8.9402)
  arc A187 (11.5604, -8.9402) -> (10.7167, -9.249) centre (11.4173, -9.8561) ccw
  line L112 (10.7167, -9.249) -> (10.6801, -9.2914)
  arc A188 (10.6801, -9.2914) -> (10.4944, -10.1704) centre (11.3806, -9.8984) ccw
  line L113 (10.4944, -10.1704) -> (10.7131, -10.883)
  arc A189 (10.663, -11.0766) -> (10.7131, -10.883) centre (10.5305, -10.939) ccw
  arc A190 (10.5567, -11.1779) -> (10.663, -11.0766) centre (0, 0) ccw
  arc A191 (10.3609, -11.2188) -> (10.5567, -11.1779) centre (10.4256, -11.0391) ccw
  line L114 (10.3609, -11.2188) -> (9.6595, -10.9665)
  arc A192 (9.6595, -10.9665) -> (8.7727, -11.1101) centre (9.3457, -11.8387) ccw
  line L115 (8.7727, -11.1101) -> (8.7286, -11.1447)
  arc A193 (8.7286, -11.1447) -> (8.38, -11.9726) centre (9.3017, -11.8733) ccw
  line L116 (8.38, -11.9726) -> (8.4599, -12.7138)
  arc A194 (8.374, -12.8944) -> (8.4599, -12.7138) centre (8.27, -12.7343) ccw
  arc A195 (8.2505, -12.9738) -> (8.374, -12.8944) centre (0, 0) ccw
  arc A196 (8.0505, -12.9769) -> (8.2505, -12.9738) centre (8.148, -12.8126) ccw
  line L117 (8.0505, -12.9769) -> (7.4095, -12.5963)
  arc A197 (7.4095, -12.5963) -> (6.5115, -12.5695) centre (6.9363, -13.3935) ccw
  line L118 (6.5115, -12.5695) -> (6.4618, -12.5952)
  arc A198 (6.4618, -12.5952) -> (5.9627, -13.3422) centre (6.8865, -13.4191) ccw
  line L119 (5.9627, -13.3422) -> (5.9009, -14.0851)
  arc A199 (5.7824, -14.2462) -> (5.9009, -14.0851) centre (5.7105, -14.0692) ccw
  arc A200 (5.6461, -14.3008) -> (5.7824, -14.2462) centre (0, 0) ccw
  arc A201 (5.4492, -14.2659) -> (5.6461, -14.3008) centre (5.576, -14.1231) ccw
  line L120 (5.4492, -14.2659) -> (4.8917, -13.771)
  arc A202 (4.8917, -13.771) -> (4.0151, -13.5747) centre (4.2762, -14.4641) ccw
  line L121 (4.0151, -13.5747) -> (3.9613, -13.5905)
  arc A203 (3.9613, -13.5905) -> (3.33, -14.2296) centre (4.2225, -14.4799) ccw
  line L122 (3.33, -14.2296) -> (3.1286, -14.9473)
  arc A204 (2.9818, -15.0831) -> (3.1286, -14.9473) centre (2.9447, -14.8957) ccw
  arc A205 (2.8376, -15.1109) -> (2.9818, -15.0831) centre (0, 0) ccw
  arc A206 (2.6508, -15.0394) -> (2.8376, -15.1109) centre (2.8024, -14.9232) ccw
  line L123 (2.6508, -15.0394) -> (2.1972, -14.4479)
  arc A207 (2.1972, -14.4479) -> (1.3735, -14.0892) centre (1.4616, -15.012) ccw
  line L124 (1.3735, -14.0892) -> (1.3177, -14.0946)
  arc A208 (1.3177, -14.0946) -> (0.5768, -14.6026) centre (1.4059, -15.0174) ccw
  line L125 (0.5768, -14.6026) -> (0.2433, -15.2693)
  arc A209 (0.0734, -15.3748) -> (0.2433, -15.2693) centre (0.0725, -15.1838) ccw
  arc A210 (-0.0734, -15.3748) -> (0.0734, -15.3748) centre (0, 0) ccw
  arc A211 (-0.2433, -15.2693) -> (-0.0734, -15.3748) centre (-0.0725, -15.1838) ccw
  line L126 (-0.2433, -15.2693) -> (-0.5768, -14.6026)
  arc A212 (-0.5768, -14.6026) -> (-1.3177, -14.0946) centre (-1.4059, -15.0174) ccw
  line L127 (-1.3177, -14.0946) -> (-1.3735, -14.0892)
  arc A213 (-1.3735, -14.0892) -> (-2.1972, -14.4479) centre (-1.4616, -15.012) ccw
  line L128 (-2.1972, -14.4479) -> (-2.6508, -15.0394)
  arc A214 (-2.8376, -15.1109) -> (-2.6508, -15.0394) centre (-2.8024, -14.9232) ccw
  arc A215 (-2.9818, -15.0831) -> (-2.8376, -15.1109) centre (0, 0) ccw
  arc A216 (-3.1286, -14.9473) -> (-2.9818, -15.0831) centre (-2.9447, -14.8957) ccw
  line L129 (-3.1286, -14.9473) -> (-3.33, -14.2296)
  arc A217 (-3.33, -14.2296) -> (-3.9613, -13.5905) centre (-4.2225, -14.4799) ccw
  line L130 (-3.9613, -13.5905) -> (-4.0151, -13.5747)
  arc A218 (-4.0151, -13.5747) -> (-4.8917, -13.771) centre (-4.2762, -14.4641) ccw
  line L131 (-4.8917, -13.771) -> (-5.4492, -14.2659)
  arc A219 (-5.6461, -14.3008) -> (-5.4492, -14.2659) centre (-5.576, -14.1231) ccw
  arc A220 (-5.7824, -14.2462) -> (-5.6461, -14.3008) centre (0, 0) ccw
  arc A221 (-5.9009, -14.0851) -> (-5.7824, -14.2462) centre (-5.7105, -14.0692) ccw
  line L132 (-5.9009, -14.0851) -> (-5.9627, -13.3422)
  arc A222 (-5.9627, -13.3422) -> (-6.4618, -12.5952) centre (-6.8865, -13.4191) ccw
  line L133 (-6.4618, -12.5952) -> (-6.5115, -12.5695)
  arc A223 (-6.5115, -12.5695) -> (-7.4095, -12.5963) centre (-6.9363, -13.3935) ccw
  line L134 (-7.4095, -12.5963) -> (-8.0505, -12.9769)
  arc A224 (-8.2505, -12.9738) -> (-8.0505, -12.9769) centre (-8.148, -12.8126) ccw
  arc A225 (-8.374, -12.8944) -> (-8.2505, -12.9738) centre (0, 0) ccw
  arc A226 (-8.4599, -12.7138) -> (-8.374, -12.8944) centre (-8.27, -12.7343) ccw
  line L135 (-8.4599, -12.7138) -> (-8.38, -11.9726)
  arc A227 (-8.38, -11.9726) -> (-8.7286, -11.1447) centre (-9.3017, -11.8733) ccw
  line L136 (-8.7286, -11.1447) -> (-8.7727, -11.1101)
  arc A228 (-8.7727, -11.1101) -> (-9.6595, -10.9665) centre (-9.3457, -11.8387) ccw
  line L137 (-9.6595, -10.9665) -> (-10.3609, -11.2188)
  arc A229 (-10.5567, -11.1779) -> (-10.3609, -11.2188) centre (-10.4256, -11.0391) ccw
  arc A230 (-10.663, -11.0766) -> (-10.5567, -11.1779) centre (0, 0) ccw
  arc A231 (-10.7131, -10.883) -> (-10.663, -11.0766) centre (-10.5305, -10.939) ccw
  line L138 (-10.7131, -10.883) -> (-10.4944, -10.1704)
  arc A232 (-10.4944, -10.1704) -> (-10.6801, -9.2914) centre (-11.3806, -9.8984) ccw
  line L139 (-10.6801, -9.2914) -> (-10.7167, -9.249)
  arc A233 (-10.7167, -9.249) -> (-11.5604, -8.9402) centre (-11.4173, -9.8561) ccw
  line L140 (-11.5604, -8.9402) -> (-12.2969, -9.0552)
  arc A234 (-12.4814, -8.9781) -> (-12.2969, -9.0552) centre (-12.3263, -8.8665) ccw
  arc A235 (-12.5665, -8.8585) -> (-12.4814, -8.9781) centre (0, 0) ccw
  arc A236 (-12.5791, -8.6589) -> (-12.5665, -8.8585) centre (-12.4104, -8.7484) ccw
  line L141 (-12.5791, -8.6589) -> (-12.2295, -8.0005)
  arc A237 (-12.2295, -8.0005) -> (-12.2455, -7.1022) centre (-13.0483, -7.5657) ccw
  line L142 (-12.2455, -7.1022) -> (-12.2735, -7.0538)
  arc A238 (-12.2735, -7.0538) -> (-13.0434, -6.5908) centre (-13.0763, -7.5173) ccw
  line L143 (-13.0434, -6.5908) -> (-13.7884, -6.5644)
  arc A239 (-13.9549, -6.4537) -> (-13.7884, -6.5644) centre (-13.7816, -6.3735) ccw
  arc A240 (-14.0159, -6.3202) -> (-13.9549, -6.4537) centre (0, 0) ccw
  arc A241 (-13.9905, -6.1218) -> (-14.0159, -6.3202) centre (-13.8418, -6.2417) ccw
  line L144 (-13.9905, -6.1218) -> (-13.5226, -5.5415)
  arc A242 (-13.5226, -5.5415) -> (-13.3683, -4.6564) centre (-14.2443, -4.9596) ccw
  line L145 (-13.3683, -4.6564) -> (-13.3866, -4.6035)
  arc A243 (-13.3866, -4.6035) -> (-14.055, -4.0033) centre (-14.2626, -4.9067) ccw
  line L146 (-14.055, -4.0033) -> (-14.7815, -3.8363)
  arc A244 (-14.9241, -3.6961) -> (-14.7815, -3.8363) centre (-14.7387, -3.6502) ccw
  arc A245 (-14.9587, -3.5534) -> (-14.9241, -3.6961) centre (0, 0) ccw
  arc A246 (-14.8962, -3.3634) -> (-14.9587, -3.5534) centre (-14.7729, -3.5093) ccw
  line L147 (-14.8962, -3.3634) -> (-14.327, -2.8821)
  arc A247 (-14.327, -2.8821) -> (-14.0079, -2.0423) centre (-14.9255, -2.1742) ccw
  line L148 (-14.0079, -2.0423) -> (-14.0159, -1.9869)
  arc A248 (-14.0159, -1.9869) -> (-14.5586, -1.271) centre (-14.9335, -2.1188) ccw
  line L149 (-14.5586, -1.271) -> (-15.2404, -0.9696)
  arc A249 (-15.3539, -0.8049) -> (-15.2404, -0.9696) centre (-15.1632, -0.7949) ccw
  arc A250 (-15.3609, -0.6583) -> (-15.3539, -0.8049) centre (0, 0) ccw
  arc A251 (-15.2636, -0.4835) -> (-15.3609, -0.6583) centre (-15.1701, -0.6501) ccw
  line L150 (-15.2636, -0.4835) -> (-14.6135, -0.1187)
  arc A252 (-14.6135, -0.1187) -> (-14.1413, 0.6456) centre (-15.0672, 0.6897) ccw
  line L151 (-14.1413, 0.6456) -> (-14.1386, 0.7015)
  arc A253 (-14.1386, 0.7015) -> (-14.5361, 1.5072) centre (-15.0646, 0.7456) ccw
  line L152 (-14.5361, 1.5072) -> (-15.1485, 1.9322)
  arc A254 (-15.2288, 2.1154) -> (-15.1485, 1.9322) centre (-15.0396, 2.0891) ccw
  arc A255 (-15.2079, 2.2607) -> (-15.2288, 2.1154) centre (0, 0) ccw
  arc A256 (-15.0792, 2.4139) -> (-15.2079, 2.2607) centre (-15.019, 2.2326) ccw
  line L153 (-15.0792, 2.4139) -> (-14.3719, 2.6491)
  arc A257 (-14.3719, 2.6491) -> (-13.7636, 3.3102) centre (-14.6644, 3.5287) ccw
  line L154 (-13.7636, 3.3102) -> (-13.7504, 3.3646)
  arc A258 (-13.7504, 3.3646) -> (-13.9881, 4.231) centre (-14.6512, 3.5832) ccw
  line L155 (-13.9881, 4.231) -> (-14.5091, 4.7642)
  arc A259 (-14.5532, 4.9593) -> (-14.5091, 4.7642) centre (-14.3724, 4.8977) ccw
  arc A260 (-14.5052, 5.098) -> (-14.5532, 4.9593) centre (0, 0) ccw
  arc A261 (-14.3499, 5.224) -> (-14.5052, 5.098) centre (-14.325, 5.0346) ccw
  line L156 (-14.3499, 5.224) -> (-13.6108, 5.3211)
  arc A262 (-13.6108, 5.3211) -> (-12.8884, 5.8551) centre (-13.7316, 6.2402) ccw
  line L157 (-12.8884, 5.8551) -> (-12.8651, 5.9061)
  arc A263 (-12.8651, 5.9061) -> (-12.9346, 6.8018) centre (-13.7083, 6.2912) ccw
  line L158 (-12.9346, 6.8018) -> (-13.3452, 7.4239)
  arc A264 (-13.3517, 7.6239) -> (-13.3452, 7.4239) centre (-13.1858, 7.5291) ccw
  arc A265 (-13.2783, 7.751) -> (-13.3517, 7.6239) centre (0, 0) ccw
  arc A266 (-13.1019, 7.8453) -> (-13.2783, 7.751) centre (-13.1133, 7.6547) ccw
  line L159 (-13.1019, 7.8453) -> (-12.3578, 7.8008)
  arc A267 (-12.3578, 7.8008) -> (-11.5474, 8.1885) centre (-12.3025, 8.7262) ccw
  line L160 (-11.5474, 8.1885) -> (-11.5149, 8.2341)
  arc A268 (-11.5149, 8.2341) -> (-11.4137, 9.1267) centre (-12.27, 8.7718) ccw
  line L161 (-11.4137, 9.1267) -> (-11.6991, 9.8154)
  arc A269 (-11.6676, 10.0129) -> (-11.6991, 9.8154) centre (-11.5226, 9.8885) ccw
  arc A270 (-11.5715, 10.1238) -> (-11.6676, 10.0129) centre (0, 0) ccw
  arc A271 (-11.3804, 10.1831) -> (-11.5715, 10.1238) centre (-11.4277, 9.9981) ccw
  line L162 (-11.3804, 10.1831) -> (-10.6582, 9.9986)
  arc A272 (-10.6582, 9.9986) -> (-9.789, 10.2259) centre (-10.4287, 10.8968) ccw
  line L163 (-9.789, 10.2259) -> (-9.7485, 10.2645)
  arc A273 (-9.7485, 10.2645) -> (-9.4801, 11.1219) centre (-10.3882, 10.9354) ccw
  line L164 (-9.4801, 11.1219) -> (-9.6301, 11.8521)
  arc A274 (-9.5618, 12.0401) -> (-9.6301, 11.8521) centre (-9.443, 11.8905) ccw
  arc A275 (-9.4464, 12.1308) -> (-9.5618, 12.0401) centre (0, 0) ccw
  arc A276 (-9.2476, 12.1529) -> (-9.4464, 12.1308) centre (-9.329, 11.9801) ccw
  line L165 (-9.2476, 12.1529) -> (-8.5733, 11.835)
  arc A277 (-8.5733, 11.835) -> (-7.6769, 11.8936) centre (-8.178, 12.6735) ccw
  line L166 (-7.6769, 11.8936) -> (-7.6298, 11.9239)
  arc A278 (-7.6298, 11.9239) -> (-7.204, 12.715) centre (-8.1309, 12.7038) ccw
  line L167 (-7.204, 12.715) -> (-7.213, 13.4604)
  arc A279 (-7.1104, 13.6321) -> (-7.213, 13.4604) centre (-7.0221, 13.4627) ccw
  arc A280 (-6.9799, 13.6993) -> (-7.1104, 13.6321) centre (0, 0) ccw
  arc A281 (-6.7805, 13.6834) -> (-6.9799, 13.6993) centre (-6.8932, 13.5291) ccw
  line L168 (-6.7805, 13.6834) -> (-6.1786, 13.2436)
  arc A282 (-6.1786, 13.2436) -> (-5.2872, 13.1316) centre (-5.6318, 13.9922) ccw
  line L169 (-5.2872, 13.1316) -> (-5.2353, 13.1524)
  arc A283 (-5.2353, 13.1524) -> (-4.6675, 13.8486) centre (-5.5798, 14.013) ccw
  line L170 (-4.6675, 13.8486) -> (-4.5353, 14.5822)
  arc A284 (-4.402, 14.7314) -> (-4.5353, 14.5822) centre (-4.3473, 14.5484) ccw
  arc A285 (-4.2612, 14.7727) -> (-4.402, 14.7314) centre (0, 0) ccw
  arc A286 (-4.0684, 14.7193) -> (-4.2612, 14.7727) centre (-4.2082, 14.5892) ccw
  line L171 (-4.0684, 14.7193) -> (-3.5606, 14.1736)
  arc A287 (-3.5606, 14.1736) -> (-2.7065, 13.8949) centre (-2.882, 14.8051) ccw
  line L172 (-2.7065, 13.8949) -> (-2.6515, 13.9055)
  arc A288 (-2.6515, 13.9055) -> (-1.9623, 14.4817) centre (-2.827, 14.8157) ccw
  line L173 (-1.9623, 14.4817) -> (-1.6936, 15.177)
  arc A289 (-1.5345, 15.2982) -> (-1.6936, 15.177) centre (-1.5155, 15.1082) ccw
  arc A290 (-1.3884, 15.3122) -> (-1.5345, 15.2982) centre (0, 0) ccw
  arc A291 (-1.2092, 15.2233) -> (-1.3884, 15.3122) centre (-1.3712, 15.122) ccw
  line L174 (-1.2092, 15.2233) -> (-0.8139, 14.5913)
  arc A292 (-0.8139, 14.5913) -> (-0.028, 14.156) centre (-0.028, 15.083) ccw
  line L175 (-0.028, 14.156) -> (0.028, 14.156)
  arc A293 (0.028, 14.156) -> (0.8139, 14.5913) centre (0.028, 15.083) ccw
  line L176 (0.8139, 14.5913) -> (1.2092, 15.2233)
  arc A294 (1.3884, 15.3122) -> (1.2092, 15.2233) centre (1.3712, 15.122) ccw
  arc A295 (1.5345, 15.2982) -> (1.3884, 15.3122) centre (0, 0) ccw
  arc A296 (1.6936, 15.177) -> (1.5345, 15.2982) centre (1.5155, 15.1082) ccw
  line L177 (1.6936, 15.177) -> (1.9623, 14.4817)
  arc A297 (1.9623, 14.4817) -> (2.6515, 13.9055) centre (2.827, 14.8157) ccw
  line L178 (2.6515, 13.9055) -> (2.7065, 13.8949)
  arc A298 (2.7065, 13.8949) -> (3.5606, 14.1736) centre (2.882, 14.8051) ccw
  line L179 (3.5606, 14.1736) -> (4.0684, 14.7193)
  arc A299 (4.2612, 14.7727) -> (4.0684, 14.7193) centre (4.2082, 14.5892) ccw
  arc A300 (4.402, 14.7314) -> (4.2612, 14.7727) centre (0, 0) ccw
  arc A301 (4.5353, 14.5822) -> (4.402, 14.7314) centre (4.3473, 14.5484) ccw
  line L180 (4.5353, 14.5822) -> (4.6675, 13.8486)
  arc A302 (4.6675, 13.8486) -> (5.2353, 13.1524) centre (5.5798, 14.013) ccw
  line L181 (5.2353, 13.1524) -> (5.2872, 13.1316)
  arc A303 (5.2872, 13.1316) -> (6.1786, 13.2436) centre (5.6318, 13.9922) ccw
  line L182 (6.1786, 13.2436) -> (6.7805, 13.6834)
  arc A304 (6.9799, 13.6993) -> (6.7805, 13.6834) centre (6.8932, 13.5291) ccw
  arc A305 (7.1104, 13.6321) -> (6.9799, 13.6993) centre (0, 0) ccw
  arc A306 (7.213, 13.4604) -> (7.1104, 13.6321) centre (7.0221, 13.4627) ccw
  line L183 (7.213, 13.4604) -> (7.204, 12.715)
  arc A307 (7.204, 12.715) -> (7.6298, 11.9239) centre (8.1309, 12.7038) ccw
  line L184 (7.6298, 11.9239) -> (7.6769, 11.8936)
  arc A308 (7.6769, 11.8936) -> (8.5733, 11.835) centre (8.178, 12.6735) ccw
  line L185 (8.5733, 11.835) -> (9.2476, 12.1529)
  arc A309 (9.4464, 12.1308) -> (9.2476, 12.1529) centre (9.329, 11.9801) ccw
  arc A310 (9.5618, 12.0401) -> (9.4464, 12.1308) centre (0, 0) ccw
  arc A311 (9.6301, 11.8521) -> (9.5618, 12.0401) centre (9.443, 11.8905) ccw
  line L186 (9.6301, 11.8521) -> (9.4801, 11.1219)
  arc A312 (9.4801, 11.1219) -> (9.7485, 10.2645) centre (10.3882, 10.9354) ccw
  line L187 (9.7485, 10.2645) -> (9.789, 10.2259)
  arc A313 (9.789, 10.2259) -> (10.6582, 9.9986) centre (10.4287, 10.8968) ccw
  line L188 (10.6582, 9.9986) -> (11.3804, 10.1831)
  arc A314 (11.5715, 10.1238) -> (11.3804, 10.1831) centre (11.4277, 9.9981) ccw
  arc A315 (11.6676, 10.0129) -> (11.5715, 10.1238) centre (0, 0) ccw
  arc A316 (11.6991, 9.8154) -> (11.6676, 10.0129) centre (11.5226, 9.8885) ccw
  line L189 (11.6991, 9.8154) -> (11.4137, 9.1267)
  arc A317 (11.4137, 9.1267) -> (11.5149, 8.2341) centre (12.27, 8.7718) ccw
  line L190 (11.5149, 8.2341) -> (11.5474, 8.1885)
  arc A318 (11.5474, 8.1885) -> (12.3578, 7.8008) centre (12.3025, 8.7262) ccw
  line L191 (12.3578, 7.8008) -> (13.1019, 7.8453)
  arc A319 (13.2783, 7.751) -> (13.1019, 7.8453) centre (13.1133, 7.6547) ccw
  arc A320 (13.3517, 7.6239) -> (13.2783, 7.751) centre (0, 0) ccw
  arc A321 (13.3452, 7.4239) -> (13.3517, 7.6239) centre (13.1858, 7.5291) ccw
  line L192 (13.3452, 7.4239) -> (12.9346, 6.8018)
  arc A322 (12.9346, 6.8018) -> (12.8651, 5.9061) centre (13.7083, 6.2912) ccw
  line L193 (12.8651, 5.9061) -> (12.8884, 5.8551)
  arc A323 (12.8884, 5.8551) -> (13.6108, 5.3211) centre (13.7316, 6.2402) ccw
  line L194 (13.6108, 5.3211) -> (14.3499, 5.224)
  arc A324 (14.5052, 5.098) -> (14.3499, 5.224) centre (14.325, 5.0346) ccw
  arc A325 (14.5532, 4.9593) -> (14.5052, 5.098) centre (0, 0) ccw
  arc A326 (14.5091, 4.7642) -> (14.5532, 4.9593) centre (14.3724, 4.8977) ccw
  line L195 (14.5091, 4.7642) -> (13.9881, 4.231)
  arc A327 (13.9881, 4.231) -> (13.7504, 3.3646) centre (14.6512, 3.5832) ccw
  line L196 (13.7504, 3.3646) -> (13.7636, 3.3102)
  arc A328 (13.7636, 3.3102) -> (14.3719, 2.6491) centre (14.6644, 3.5287) ccw
  line L197 (14.3719, 2.6491) -> (15.0792, 2.4139)
  arc A329 (15.2079, 2.2607) -> (15.0792, 2.4139) centre (15.019, 2.2326) ccw
  line L198 (0, -22.75) -> (0, 22.75) construction
  line L199 (-22.75, 0) -> (22.75, 0) construction
  circle A330 centre (0, 0) radius 1.5
  circle A331 centre (0, 0) radius 15.75
  circle A332 centre (0, 0) radius 16.25
  dimension "d54" = 3
  dimension "d55" = 31.5